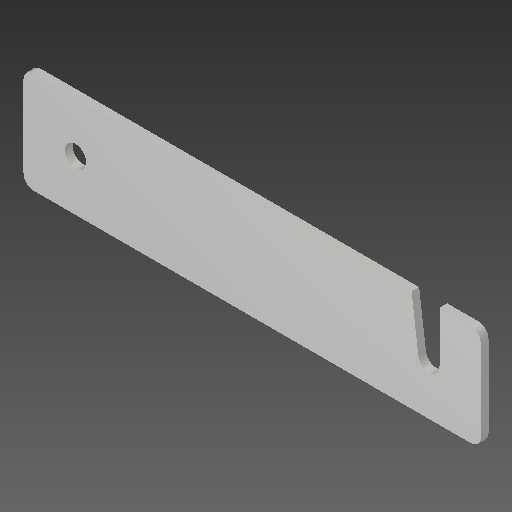
# Autodesk Inventor part: 3d_LM-Welding_Tooling -  Tab
Saved by Autodesk Inventor 2018.3 (Build 223284000, 284)
## iProperties
Created: 2026-01-29
Part Number: 3d_LM-Welding_Tooling -  Tab
Material: Aluminium 6061-T6
Document SubType Name: Sheet Metal
Designer: aca6
Density: 2.7 g/cm^3
Appearance: N/A - Machined Aluminium
Sheet Metal Rule: Default_mm
Manufacturer-1: {"Name": "Hanstar Technologies Co., Ltd", "PartNumber": "3d_Welding_Tooling -  Tab", "Link": ""}
Manufacturer-2: {"Name": "SHENZHEN JINYIHE PROTOTYPE TECHNOLOGIES CO., LTD", "PartNumber": "3d_Welding_Tooling -  Tab", "Link": ""}
Manufacturer-3: {"Name": "Shenzhen city Xavier Precision Co., Ltd.", "PartNumber": "3d_Welding_Tooling -  Tab", "Link": ""}
Manufacturer-4: {"Name": "", "PartNumber": "", "Link": ""}
Manufacturer-5: {"Name": "", "PartNumber": "", "Link": ""}
Provider-1: {"Name": "", "PartNumber": "", "Link": ""}
Provider-2: {"Name": "", "PartNumber": "", "Link": ""}
Provider-3: {"Name": "", "PartNumber": "", "Link": ""}
Provider-4: {"Name": "", "PartNumber": "", "Link": ""}
Provider-5: {"Name": "", "PartNumber": "", "Link": ""}
Author: aca6
Comments: DIN-ISO-2768-mK
Autodesk Inventor part; units mm, degrees
ref_plane "YZ Plane" through (0, 0, 0) normal (1, 0, 0) x (0, 1, 0)
ref_plane "XZ Plane" through (0, 0, 0) normal (0, 1, 0) x (-1, 0, 0)
ref_plane "XY Plane" through (0, 0, 0) normal (0, 0, 1) x (1, 0, 0)
sketch "Sketch1" plane through (0, 0, 0) normal (0, 0, 1) x (1, 0, 0)
  line L0 (-45, 10) -> (45, 10)
  line L1 (45, 10) -> (45, -10)
  line L2 (45, -10) -> (-45, -10)
  line L3 (-45, -10) -> (-45, 10)
  line L4 (0, 0) -> (0, 7.2508) construction
  line L5 (0, 0) -> (8.0596, 0) construction
  dimension "d0" = 90
  dimension "d1" = 20
  measures "d0" distance of L0.start L0.end
  measures "d1" distance of L0.end L1.end
extrude "Plate1" add sketch "Sketch1" along normal blind 1.5
fillet "Fillet1" radius 2 4 edges at (45, 10, 0.75) (45, -10, 0.75) (-45, -10, 0.75) (-45, 10, 0.75)
sketch "Sketch2" plane through (0, 0, 1.5) normal (0, 0, 1) x (1, 0, 0)
  line L0 (-45, -8) -> (-45, 8) projected
  line L1 (45, 8) -> (45, -8) projected
  arc A0 (32.65, 0) -> (36.85, 0) centre (34.75, 0) ccw
  line L2 (36.85, 0) -> (36.85, 10)
  line L3 (32.65, 0) -> (32.65, 10)
  line L4 (43, -10) -> (-43, -10) projected
  line L5 (-43, 10) -> (43, 10) projected
  point P0 (0, 0)
  dimension "d5" = 10.25
  dimension "d6" = 4.2
  dimension "d7" = 10
  constraints: 4 end point, 2 point on circle, 2 point on line, 2 tangent, 2 vertical, 1 centre point, 1 coincident
  measures "d5" distance from line of L1 point (34.75, 0)
  measures "d6" diameter of A0
  measures "d7" distance from line of L4 point (34.75, 0)
extrude "Cut1" cut sketch "Sketch2" against normal blind 1.5
sketch "Sketch3" plane through (0, 0, 1.5) normal (0, 0, 1) x (1, 0, 0)
  line L0 (-45, -8) -> (-45, 8) projected
  point P0 (0, 0)
  point P1 (-34.75, 0)
  dimension "d10" = 10.25
  constraints: 1 horizontal alignment
  measures "d10" distance from line of L0 point (-34.75, 0)
hole "Hole1" at (-34.75, 0, 1.5) direction (0, 0, -1) diameter 4.2 depth 1.5 tip angle 118
sketch "Sketch5" plane through (0, 0, 1.5) normal (0, 0, 1) x (1, 0, 0)
  circle A0 centre (34.0345, 9.9478) radius 2.121 projected
  arc A1 (32.65, 0) -> (36.85, 0) centre (34.75, 0) ccw projected
  line L0 (34.75, 0) -> (34.0345, 9.9478)
  line L1 (32.65, 0) -> (31.9141, 10)
  line L2 (-43, 10) -> (32.65, 10) projected
  line L3 (36.85, 0) -> (36.1504, 10.0945)
  line L4 (32.65, 0) -> (32.65, 10) projected
  line L5 (32.65, 0) -> (32.65, 10)
  line L6 (32.65, 10) -> (31.9141, 10)
  line L7 (32.65, 10) -> (32.65, 0) projected
  line L8 (32.65, 0) -> (31.35, 10)
  line L9 (-43, 10) -> (32.65, 10) projected
  line L10 (31.35, 10) -> (32.65, 10)
  point P0 (0, 0)
  dimension "d20" = 1.3
  constraints: 14 end point, 2 collinear, 2 point on circle, 2 point on line, 1 perpendicular, 1 tangent
  measures "d20" distance of L2.end L8.end
extrude "Cut2" cut sketch "Sketch5" against normal blind 1.5 contours L1 A0 | L2 L4 A0 L1 | A0 L1 L8 L2 | L4 L1 A0
equation "\"d8\" = Thickness"
equation "\"d16\" = Thickness"
equation "\"d18\" = Thickness"
equation "\"d2\" = Thickness"
equation "\"BendRadius\" = Thickness"
equation "\"BendReliefWidth\" = Thickness"
equation "\"BendReliefDepth\" = 0.5 * Thickness"
equation "\"CornerReliefSize\" = 4 * Thickness"
equation "\"MinimumRemnant\" = 2 * Thickness"
equation "\"TransitionRadius\" = BendRadius"
equation "\"JacobiRadiusSize\" = BendRadius"
equation "\"GapSize\" = Thickness"
equation "\"Thickness\" = 1.5"
body "Solid1"
